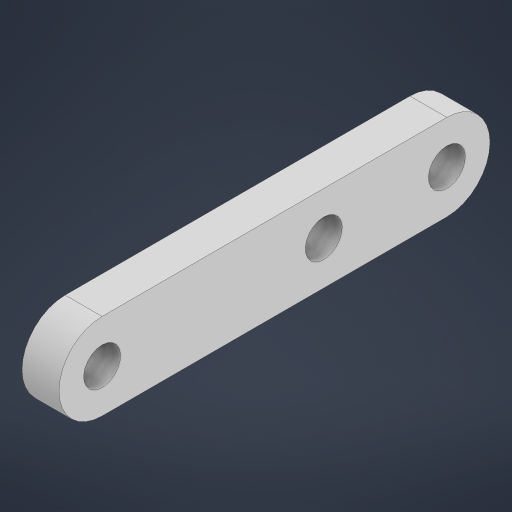
# Autodesk Inventor part: acople_gripper
Saved by Autodesk Inventor 2023.1 (Build 271208000, 208)
## iProperties
Created: 2022-10-23
Part Number: acople_gripper
Material: Generic
Document SubType Name: Modeling
Designer: amtat
Density: 1 g/cm^3
Appearance: Default
Author: amtat
Autodesk Inventor part; units mm, degrees
ref_plane "YZ Plane" through (0, 0, 0) normal (1, 0, 0) x (0, 1, 0)
ref_plane "XZ Plane" through (0, 0, 0) normal (0, 1, 0) x (-1, 0, 0)
ref_plane "XY Plane" through (0, 0, 0) normal (0, 0, 1) x (1, 0, 0)
sketch "Sketch1" plane through (0, 0, 0) normal (1, 0, 0) x (0, 1, 0)
  circle A0 centre (0, 0) radius 1.5
  arc A1 (3.5, 0) -> (0, -3.5) centre (0, 0) ccw
  line L0 (0, 0) -> (0, -18)
  circle A2 centre (0, -18) radius 1.5
  line L1 (0, -18) -> (0, -28)
  circle A3 centre (0, -28) radius 1.5
  arc A4 (0, -24.5) -> (3.5, -28) centre (0, -28) ccw
  line L2 (3.5, 0) -> (3.5, -28)
  line L3 (-3.5, 0) -> (-3.5, -28)
  dimension "d0" = 3
  dimension "d1" = 7
  dimension "d2" = 18
  dimension "d3" = 3
  dimension "d4" = 10
  dimension "d5" = 3
  dimension "d6" = 7
  constraints: 8 end point, 6 point on circle, 5 centre point, 5 coincident, 2 point on line, 2 tangent, 2 vertical
  measures "d0" diameter of A0
  measures "d1" diameter of A1
  measures "d2" distance of L0.start L0.end
  measures "d3" diameter of A2
  measures "d4" distance of L1.start L1.end
  measures "d5" diameter of A3
  measures "d6" diameter of A4
extrude "Extrusion1" add sketch "Sketch1" along normal blind 3 contours A1 L2 A4 L1 A2 L0 | L0 A2 L1 A4 L3 A1
body "Solid1"
